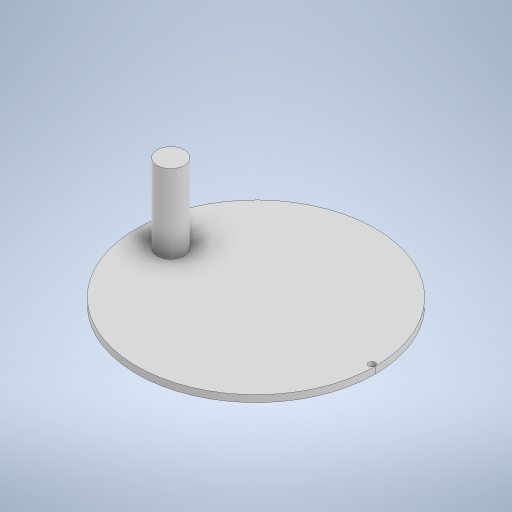
# Autodesk Inventor part: Feul_ClosePlate
Saved by Autodesk Inventor 2024.3 (Build 283343000, 343)
## iProperties
Created: 2025-03-09
Part Number: Feul_ClosePlate
Material: Generic
Document SubType Name: Modeling
Designer: ajclo
Density: 1 g/cm^3
Appearance: Default
Author: ajclo
Autodesk Inventor part; units mm, degrees
ref_plane "YZ Plane" through (0, 0, 0) normal (1, 0, 0) x (0, 1, 0)
ref_plane "XZ Plane" through (0, 0, 0) normal (0, 1, 0) x (-1, 0, 0)
ref_plane "XY Plane" through (0, 0, 0) normal (0, 0, 1) x (1, 0, 0)
sketch "Sketch1" plane through (0, 0, 0) normal (0, 1, 0) x (-1, 0, 0)
  circle A0 centre (0, 0) radius 35
  circle A1 centre (25, 0) radius 4
  dimension "d0" = 70
  dimension "d1" = 8
  dimension "d2" = 25
  constraints: 2 centre point, 1 coincident
  measures "d0" diameter of A0
  measures "d1" diameter of A1
  measures "d2" distance of point (0, 0) A1.centre
extrude "Extrusion1" add sketch "Sketch1" along normal blind 2
extrude "Extrusion2" add sketch "Sketch1" along normal blind 25 contours A1
sketch "Sketch2" plane through (0, 2, 0) normal (0, 1, 0) x (1, 0, 0)
  point P0 (0, 0)
sketch "Sketch3" plane through (0, 2, 0) normal (0, 1, 0) x (1, 0, 0)
  circle A0 centre (34, 0) radius 1
  point P0 (0, 0)
  dimension "d7" = 2
  dimension "d8" = 34
  constraints: 1 centre point
  measures "d7" diameter of A0
  measures "d8" distance of point (0, 0) A0.centre
extrude "Extrusion3" cut sketch "Sketch3" against normal through all
body "Solid1"
